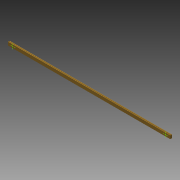
# Autodesk Inventor part: relsa2
Saved by Autodesk Inventor 2015 (Build 190159000, 159)
## iProperties
Created: 2016-04-26
Part Number: relsa2
Material: Brass, Soft Yellow
Document SubType Name: Modeling
Designer: Kostya
Density: 8.47 g/cm^3
Appearance: Brass - Satin
Author: Kostya
Autodesk Inventor part; units mm, degrees
ref_plane "YZ Plane" through (0, 0, 0) normal (1, 0, 0) x (0, 1, 0)
ref_plane "XZ Plane" through (0, 0, 0) normal (0, 1, 0) x (-1, 0, 0)
ref_plane "XY Plane" through (0, 0, 0) normal (0, 0, 1) x (1, 0, 0)
sketch "Sketch1" plane through (0, 0, 0) normal (0, 1, 0) x (-1, 0, 0)
  line L0 (0, 0) -> (0, -10)
  line L1 (0, -10) -> (500, -10)
  line L2 (500, -10) -> (500, 0)
  line L3 (500, 0) -> (0, 0)
  dimension "d0" = 10
  dimension "d1" = 500
  dimension "d2" = 500
  constraints: 8 end point, 2 perpendicular, 2 vertical
  measures "d0" distance of L0.start L0.end
  measures "d1" distance of L0.end L1.end
  measures "d2" distance of L2.end L0.start
extrude "Extrusion1" add sketch "Sketch1" along normal blind 5
sketch "Sketch5" plane through (0, 0, 0) normal (1, 0, 0) x (0, 0, -1)
  line L0 (1, 3) -> (0, 3)
  line L1 (0, 3) -> (0, 2)
  line L2 (0, 2) -> (1, 2)
  line L3 (1, 2) -> (1, 3)
  line L4 (10, 3) -> (9, 3)
  line L5 (9, 3) -> (9, 2)
  line L6 (9, 2) -> (10, 2)
  line L7 (10, 2) -> (10, 3)
  line L8 (10, 0) -> (10, 5) projected
  line L9 (0, 0) -> (0, 5) projected
  point P0 (10, 2.5)
  point P1 (0, 2.5)
  point P2 (10, 2.5)
  point P3 (0, 2.5)
  dimension "d33" = 1
  dimension "d34" = 1
  dimension "d35" = 1
  dimension "d36" = 1
  dimension "d37" = 1
  dimension "d38" = 1
  dimension "d39" = 1
  constraints: 16 end point, 4 midpoint, 4 perpendicular, 2 coincident, 2 horizontal, 2 vertical alignment
  measures "d33" distance of L0.start L0.end
  measures "d34" distance of L0.end L1.end
  measures "d35" distance of L1.end L2.end
  measures "d36" distance of L2.end L0.start
  measures "d37" distance of L4.start L4.end
  measures "d38" distance of L4.end L5.end
  measures "d39" distance of L5.end L6.end
extrude "Extrusion2" cut sketch "Sketch5" against normal up to next
sketch "Sketch7" plane through (0, 0, 0) normal (0, -1, 0) x (1, 0, 0)
  circle A0 centre (-11, -5) radius 1.5
  circle A1 centre (-490, -5) radius 1.5
  line L0 (-500, -10) -> (-500, 0) projected
  point P0 (0, 0)
  dimension "d42" = 3
  dimension "d43" = 3
  dimension "d44" = 479
  dimension "d45" = 10
  constraints: 2 centre point
  measures "d42" diameter of A0
  measures "d43" diameter of A1
  measures "d44" distance of A1.centre A0.centre
  measures "d45" distance from line of L0 A1.centre
extrude "Extrusion3" cut sketch "Sketch7" against normal up to next
sketch "Sketch2" plane through (0, 0, 0) normal (0, -1, 0) x (1, 0, 0)
  point P0 (-485, -5)
sketch "Sketch3" plane through (0, 0, 0) normal (0, -1, 0) x (1, 0, 0)
  point P0 (-15, -5)
body "Solid1"
